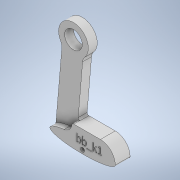
# Autodesk Inventor part: passive_walking_robot1
Saved by Autodesk Inventor 2021 (Build 250183000, 183)
## iProperties
Created: 2024-05-30
Part Number: passive_walking_robot1
Material: 一般
Document SubType Name: Modeling
Designer: 山下　響
Density: 1 g/cm^3
Appearance: 既定
Author: 山下　響
Autodesk Inventor part; units mm, degrees
ref_plane "YZ Plane" through (0, 0, 0) normal (1, 0, 0) x (0, 1, 0)
ref_plane "XZ Plane" through (0, 0, 0) normal (0, 1, 0) x (-1, 0, 0)
ref_plane "XY Plane" through (0, 0, 0) normal (0, 0, 1) x (1, 0, 0)
sketch "スケッチ1" plane through (0, 0, 0) normal (0, 0, 1) x (1, 0, 0)
  point P0 (0, 0)
sketch "スケッチ2" plane through (0, 0, 0) normal (0, 0, 1) x (1, 0, 0)
  line L0 (0, 0) -> (110, 0)
  line L1 (110, 0) -> (110, -25)
  line L2 (110, -25) -> (0, -25)
  line L3 (0, -25) -> (0, 0)
  ellipse E0 centre (55, -25) end of major axis (110, -25) minor radius 11.2287
  line L4 (0, -25) -> (13.9449, 134.3912)
  line L5 (13.9449, 134.3912) -> (48.8117, 131.3407)
  line L6 (48.8117, 131.3407) -> (34.8668, -28.0505)
  line L7 (34.8668, -28.0505) -> (0, -25)
  circle A0 centre (29.6352, 112.942) radius 14.8
  circle A1 centre (29.6352, 112.942) radius 25
  point P0 (0.0351, -24.599)
  point P1 (36.056, -14.4584)
  point P2 (37.3209, 0)
  dimension "d0" = 110
  dimension "d1" = 25
  dimension "d2" = 35
  dimension "d4" = 160
  dimension "d5" = 5
  dimension "d6" = 29.6
  dimension "d7" = 17.5
  dimension "d18" = 20
  dimension "d23" = 50
  constraints: 16 end point, 4 parallel, 2 centre point, 2 horizontal, 2 perpendicular, 1 coincident, 1 midpoint, 3 other
  measures "d0" distance of L1.end L2.end
  measures "d1" distance of L0.end L1.end
  measures "d2" distance of L4.end L5.end
  measures "d4" distance between parallel lines of L5 L7
  measures "d5" angle of L3 L4
  measures "d6" diameter of A0
  measures "d7" distance from line of L4 A0.centre
  measures "d18" distance from line of L5 A0.centre
  measures "d23" diameter of A1
extrude "押し出し1" add sketch "スケッチ2" along normal blind 15 contours L4 A1 L6 L0 | L0 L6 E0 L4 | L4 A1 L5 L6 | L4 L5 A1 | A1 L5 L6
extrude "押し出し2" add sketch "スケッチ2" along normal blind 25 contours L4 E0 L6 L2 | L7 L6 L2 E0 | E0 L4 | L2 L6 L7 | L0 L1 E0 L6 | L6 E0 L2
fillet "フィレット1" radius 3 2 edges at (37.3209, 0, 20) (37.3209, 0, 7.5)
fillet "フィレット2" radius 25 1 edges at (110, 0, 12.5)
fillet "フィレット3" radius 15 2 edges at (48.8117, 131.3407, 7.5) (13.9449, 134.3912, 7.5)
fillet "フィレット4" radius 15 1 edges at (36.056, -14.4584, 20)
sketch "スケッチ3" plane through (0, 0, 25) normal (0, 0, 1) x (1, 0, 0)
  line L0 (43.9254, -10.4065) -> (55.2208, -10.4065) construction
  line L1 (55.2208, -10.4065) -> (55.2208, -14.2029) construction
  line L2 (55.2208, -14.2029) -> (43.9254, -14.2029) construction
  line L3 (43.9254, -14.2029) -> (43.9254, -10.4065) construction
  spline S0 degree 2 poles (52.5705, -18.2931) (52.5705, -20.5005) (50.4311, -23.1942) (48.8168, -23.1942) knots 0 0 0 1 2 2 2
  spline S1 degree 2 poles (48.8168, -23.1942) (48.0875, -23.1942) (47.047, -22.8344) (46.5413, -22.5232) knots 0 0 0 1 2 2 2
  line L4 (46.5413, -22.5232) -> (46.444, -22.9414)
  line L5 (46.444, -22.9414) -> (45.0243, -22.9414)
  line L6 (45.0243, -22.9414) -> (45.0243, -10.4065)
  line L7 (45.0243, -10.4065) -> (46.5413, -10.4065)
  line L8 (46.5413, -10.4065) -> (46.5413, -14.8798)
  spline S2 degree 2 poles (46.5413, -14.8798) (47.115, -14.3644) (48.4473, -13.6837) (49.2933, -13.6837) knots 0 0 0 1 2 2 2
  spline S3 degree 2 poles (49.2933, -13.6837) (50.8201, -13.6837) (52.5705, -16.1245) (52.5705, -18.2931) knots 0 0 0 1 2 2 2
  spline S4 degree 2 poles (51.0048, -18.4098) (51.0048, -16.7955) (50.0226, -15.1229) (48.9335, -15.1229) knots 0 0 0 1 2 2 2
  spline S5 degree 2 poles (48.9335, -15.1229) (48.3209, -15.1229) (47.0567, -15.7064) (46.5413, -16.1537) knots 0 0 0 1 2 2 2
  line L9 (46.5413, -16.1537) -> (46.5413, -21.3174)
  spline S6 degree 2 poles (46.5413, -21.3174) (47.115, -21.5994) (48, -21.8328) (48.5251, -21.8328) knots 0 0 0 1 2 2 2
  spline S7 degree 2 poles (48.5251, -21.8328) (49.6823, -21.8328) (51.0048, -20.1893) (51.0048, -18.4098) knots 0 0 0 1 2 2 2
  spline S8 degree 2 poles (61.692, -18.2931) (61.692, -20.5005) (59.5526, -23.1942) (57.9384, -23.1942) knots 0 0 0 1 2 2 2
  spline S9 degree 2 poles (57.9384, -23.1942) (57.209, -23.1942) (56.1685, -22.8344) (55.6628, -22.5232) knots 0 0 0 1 2 2 2
  line L10 (55.6628, -22.5232) -> (55.5656, -22.9414)
  line L11 (55.5656, -22.9414) -> (54.1458, -22.9414)
  line L12 (54.1458, -22.9414) -> (54.1458, -10.4065)
  line L13 (54.1458, -10.4065) -> (55.6628, -10.4065)
  line L14 (55.6628, -10.4065) -> (55.6628, -14.8798)
  spline S10 degree 2 poles (55.6628, -14.8798) (56.2366, -14.3644) (57.5688, -13.6837) (58.4149, -13.6837) knots 0 0 0 1 2 2 2
  spline S11 degree 2 poles (58.4149, -13.6837) (59.9416, -13.6837) (61.692, -16.1245) (61.692, -18.2931) knots 0 0 0 1 2 2 2
  spline S12 degree 2 poles (60.1264, -18.4098) (60.1264, -16.7955) (59.1442, -15.1229) (58.0551, -15.1229) knots 0 0 0 1 2 2 2
  spline S13 degree 2 poles (58.0551, -15.1229) (57.4424, -15.1229) (56.1782, -15.7064) (55.6628, -16.1537) knots 0 0 0 1 2 2 2
  line L15 (55.6628, -16.1537) -> (55.6628, -21.3174)
  spline S14 degree 2 poles (55.6628, -21.3174) (56.2366, -21.5994) (57.1215, -21.8328) (57.6466, -21.8328) knots 0 0 0 1 2 2 2
  spline S15 degree 2 poles (57.6466, -21.8328) (58.8038, -21.8328) (60.1264, -20.1893) (60.1264, -18.4098) knots 0 0 0 1 2 2 2
  line L16 (71.2998, -25.353) -> (62.0421, -25.353)
  line L17 (62.0421, -25.353) -> (62.0421, -24.3125)
  line L18 (62.0421, -24.3125) -> (71.2998, -24.3125)
  line L19 (71.2998, -24.3125) -> (71.2998, -25.353)
  line L20 (79.7309, -22.9414) -> (77.7374, -22.9414)
  line L21 (77.7374, -22.9414) -> (74.3922, -18.5945)
  line L22 (74.3922, -18.5945) -> (73.7893, -19.178)
  line L23 (73.7893, -19.178) -> (73.7893, -22.9414)
  line L24 (73.7893, -22.9414) -> (72.2722, -22.9414)
  line L25 (72.2722, -22.9414) -> (72.2722, -10.4065)
  line L26 (72.2722, -10.4065) -> (73.7893, -10.4065)
  line L27 (73.7893, -10.4065) -> (73.7893, -17.7388)
  line L28 (73.7893, -17.7388) -> (77.3484, -13.9365)
  line L29 (77.3484, -13.9365) -> (79.235, -13.9365)
  line L30 (79.235, -13.9365) -> (75.5397, -17.6999)
  line L31 (75.5397, -17.6999) -> (79.7309, -22.9414)
  line L32 (87.0632, -22.9414) -> (81.209, -22.9414)
  line L33 (81.209, -22.9414) -> (81.209, -21.7161)
  line L34 (81.209, -21.7161) -> (83.3873, -21.7161)
  line L35 (83.3873, -21.7161) -> (83.3873, -13.674)
  line L36 (83.3873, -13.674) -> (81.209, -13.674)
  line L37 (81.209, -13.674) -> (81.209, -12.5751)
  spline S16 degree 2 poles (81.209, -12.5751) (82.444, -12.5751) (83.611, -11.8749) (83.6888, -10.9025) knots 0 0 0 1 2 2 2
  line L38 (83.6888, -10.9025) -> (84.9335, -10.9025)
  line L39 (84.9335, -10.9025) -> (84.9335, -21.7161)
  line L40 (84.9335, -21.7161) -> (87.0632, -21.7161)
  line L41 (87.0632, -21.7161) -> (87.0632, -22.9414)
  point P0 (0, 0)
  constraints: 2 other
extrude "押し出し3" cut sketch "スケッチ3" against normal blind 1.2
sketch "スケッチ4" plane through (0, 0, 25) normal (0, 0, 1) x (1, 0, 0)
  circle A0 centre (54.913, -30) radius 3.4
  line L0 (85, 0) -> (40.0699, 0) projected
  point P0 (0, 0)
  dimension "d19" = 6.8
  dimension "d22" = 30
  constraints: 1 centre point
  measures "d19" diameter of A0
  measures "d22" distance from line of L0 A0.centre
extrude "押し出し4" cut sketch "スケッチ4" against normal blind 40
extrude "押し出し5" add sketch "スケッチ2" along normal blind 15 contours A1 L4 | L4 A1 L5 L6 | L6 A1 | A1 L5
fillet "フィレット5" radius 15 2 edges at (45.5126, 93.6312, 7.5) (10.6458, 96.6816, 7.5)
equation "\"d7\" = 0.5 * d2"
